Autodesk Inventor part; units mm, degrees
(part 4 of 6)
  line L918 (-92.1365, -59.7341) -> (-92.1319, -59.6995) projected
  line L919 (-92.1319, -59.6995) -> (-92.1268, -59.6649) projected
  line L920 (-92.1268, -59.6649) -> (-92.121, -59.6305) projected
  line L921 (-92.121, -59.6305) -> (-92.1147, -59.5962) projected
  line L922 (-92.1147, -59.5962) -> (-92.1077, -59.562) projected
  line L923 (-92.1077, -59.562) -> (-92.1001, -59.5279) projected
  line L924 (-92.1001, -59.5279) -> (-92.092, -59.494) projected
  line L925 (-92.092, -59.494) -> (-92.0833, -59.4602) projected
  line L926 (-92.0833, -59.4602) -> (-92.0739, -59.4265) projected
  line L927 (-92.0739, -59.4265) -> (-92.064, -59.3931) projected
  line L928 (-92.064, -59.3931) -> (-92.0535, -59.3598) projected
  line L929 (-92.0535, -59.3598) -> (-92.0424, -59.3267) projected
  line L930 (-92.0424, -59.3267) -> (-92.0308, -59.2938) projected
  line L931 (-92.0308, -59.2938) -> (-92.0186, -59.2611) projected
  line L932 (-92.0186, -59.2611) -> (-92.0058, -59.2286) projected
  line L933 (-92.0058, -59.2286) -> (-91.9924, -59.1963) projected
  line L934 (-91.9924, -59.1963) -> (-91.9785, -59.1643) projected
  line L935 (-91.9785, -59.1643) -> (-91.964, -59.1326) projected
  line L936 (-91.964, -59.1326) -> (-91.949, -59.1011) projected
  line L937 (-91.949, -59.1011) -> (-91.9334, -59.0698) projected
  line L938 (-91.9334, -59.0698) -> (-91.9173, -59.0389) projected
  line L939 (-91.9173, -59.0389) -> (-91.9006, -59.0082) projected
  line L940 (-91.9006, -59.0082) -> (-91.8835, -58.9778) projected
  line L941 (-91.8835, -58.9778) -> (-91.8657, -58.9477) projected
  line L942 (-91.8657, -58.9477) -> (-91.8475, -58.918) projected
  line L943 (-91.8475, -58.918) -> (-91.8287, -58.8885) projected
  line L944 (-91.8287, -58.8885) -> (-91.8095, -58.8594) projected
  line L945 (-91.8095, -58.8594) -> (-91.7897, -58.8307) projected
  line L946 (-91.7897, -58.8307) -> (-91.7694, -58.8022) projected
  line L947 (-91.7694, -58.8022) -> (-91.7487, -58.7742) projected
  line L948 (-91.7487, -58.7742) -> (-91.7274, -58.7465) projected
  line L949 (-91.7274, -58.7465) -> (-91.7057, -58.7192) projected
  line L950 (-91.7057, -58.7192) -> (-91.6835, -58.6922) projected
  line L951 (-91.6835, -58.6922) -> (-91.6608, -58.6657) projected
  line L952 (-91.6608, -58.6657) -> (-91.6377, -58.6396) projected
  line L953 (-91.6377, -58.6396) -> (-91.6141, -58.6138) projected
  line L954 (-91.6141, -58.6138) -> (-91.5901, -58.5885) projected
  line L955 (-91.5901, -58.5885) -> (-91.5656, -58.5636) projected
  line L956 (-91.5656, -58.5636) -> (-91.5407, -58.5391) projected
  line L957 (-91.5407, -58.5391) -> (-91.5154, -58.5151) projected
  line L958 (-91.5154, -58.5151) -> (-91.4897, -58.4915) projected
  line L959 (-91.4897, -58.4915) -> (-91.4635, -58.4684) projected
  line L960 (-91.4635, -58.4684) -> (-91.437, -58.4457) projected
  line L961 (-91.437, -58.4457) -> (-91.41, -58.4235) projected
  line L962 (-91.41, -58.4235) -> (-91.3827, -58.4018) projected
  line L963 (-91.3827, -58.4018) -> (-91.355, -58.3805) projected
  line L964 (-91.355, -58.3805) -> (-91.327, -58.3598) projected
  line L965 (-91.327, -58.3598) -> (-91.2986, -58.3395) projected
  line L966 (-91.2986, -58.3395) -> (-91.2698, -58.3197) projected
  line L967 (-91.2698, -58.3197) -> (-91.2407, -58.3005) projected
  line L968 (-91.2407, -58.3005) -> (-91.2112, -58.2817) projected
  line L969 (-91.2112, -58.2817) -> (-91.1815, -58.2635) projected
  line L970 (-91.1815, -58.2635) -> (-91.1514, -58.2458) projected
  line L971 (-91.1514, -58.2458) -> (-91.121, -58.2286) projected
  line L972 (-91.121, -58.2286) -> (-91.0904, -58.2119) projected
  line L973 (-91.0904, -58.2119) -> (-91.0594, -58.1958) projected
  line L974 (-91.0594, -58.1958) -> (-91.0282, -58.1802) projected
  line L975 (-91.0282, -58.1802) -> (-90.9966, -58.1652) projected
  line L976 (-90.9966, -58.1652) -> (-90.9649, -58.1507) projected
  line L977 (-90.9649, -58.1507) -> (-90.9329, -58.1368) projected
  line L978 (-90.9329, -58.1368) -> (-90.9006, -58.1234) projected
  line L979 (-90.9006, -58.1234) -> (-90.8681, -58.1107) projected
  line L980 (-90.8681, -58.1107) -> (-90.8354, -58.0984) projected
  line L981 (-90.8354, -58.0984) -> (-90.8025, -58.0868) projected
  line L982 (-90.8025, -58.0868) -> (-90.7694, -58.0757) projected
  line L983 (-90.7694, -58.0757) -> (-90.7362, -58.0652) projected
  line L984 (-90.7362, -58.0652) -> (-90.7027, -58.0553) projected
  line L985 (-90.7027, -58.0553) -> (-90.669, -58.046) projected
  line L986 (-90.669, -58.046) -> (-90.6353, -58.0372) projected
  line L987 (-90.6353, -58.0372) -> (-90.6013, -58.0291) projected
  line L988 (-90.6013, -58.0291) -> (-90.5672, -58.0215) projected
  line L989 (-90.5672, -58.0215) -> (-90.533, -58.0146) projected
  line L990 (-90.533, -58.0146) -> (-90.4987, -58.0082) projected
  line L991 (-90.4987, -58.0082) -> (-90.4643, -58.0024) projected
  line L992 (-90.4643, -58.0024) -> (-90.4298, -57.9973) projected
  line L993 (-90.4298, -57.9973) -> (-90.3951, -57.9927) projected
  line L994 (-90.3951, -57.9927) -> (-90.3605, -57.9888) projected
  line L995 (-90.3605, -57.9888) -> (-90.3257, -57.9854) projected
  line L996 (-90.3257, -57.9854) -> (-90.2909, -57.9827) projected
  line L997 (-90.2909, -57.9827) -> (-90.2561, -57.9806) projected
  line L998 (-90.2561, -57.9806) -> (-90.2212, -57.979) projected
  line L999 (-90.2212, -57.979) -> (-90.1863, -57.9781) projected
  line L1000 (-90.1863, -57.9781) -> (-90.1514, -57.9778) projected
  line L1001 (-90.1514, -57.9778) -> (-90.1165, -57.9781) projected
  line L1002 (-90.1165, -57.9781) -> (-90.0816, -57.979) projected
  line L1003 (-90.0816, -57.979) -> (-90.0467, -57.9806) projected
  line L1004 (-90.0467, -57.9806) -> (-90.0119, -57.9827) projected
  line L1005 (-90.0119, -57.9827) -> (-89.9771, -57.9854) projected
  line L1006 (-89.9771, -57.9854) -> (-89.9424, -57.9888) projected
  line L1007 (-89.9424, -57.9888) -> (-89.9077, -57.9927) projected
  line L1008 (-89.9077, -57.9927) -> (-89.8731, -57.9973) projected
  line L1009 (-89.8731, -57.9973) -> (-89.8385, -58.0024) projected
  line L1010 (-89.8385, -58.0024) -> (-89.8041, -58.0082) projected
  line L1011 (-89.8041, -58.0082) -> (-89.7698, -58.0146) projected
  line L1012 (-89.7698, -58.0146) -> (-89.7356, -58.0215) projected
  line L1013 (-89.7356, -58.0215) -> (-89.7015, -58.0291) projected
  line L1014 (-89.7015, -58.0291) -> (-89.6676, -58.0372) projected
  line L1015 (-89.6676, -58.0372) -> (-89.6338, -58.046) projected
  line L1016 (-89.6338, -58.046) -> (-89.6001, -58.0553) projected
  line L1017 (-89.6001, -58.0553) -> (-89.5667, -58.0652) projected
  line L1018 (-89.5667, -58.0652) -> (-89.5334, -58.0757) projected
  line L1019 (-89.5334, -58.0757) -> (-89.5003, -58.0868) projected
  line L1020 (-89.5003, -58.0868) -> (-89.4674, -58.0984) projected
  line L1021 (-89.4674, -58.0984) -> (-89.4347, -58.1107) projected
  line L1022 (-89.4347, -58.1107) -> (-89.4022, -58.1234) projected
  line L1023 (-89.4022, -58.1234) -> (-89.3699, -58.1368) projected
  line L1024 (-89.3699, -58.1368) -> (-89.3379, -58.1507) projected
  line L1025 (-89.3379, -58.1507) -> (-89.3062, -58.1652) projected
  line L1026 (-89.3062, -58.1652) -> (-89.2747, -58.1802) projected
  line L1027 (-89.2747, -58.1802) -> (-89.2434, -58.1958) projected
  line L1028 (-89.2434, -58.1958) -> (-89.2125, -58.2119) projected
  line L1029 (-89.2125, -58.2119) -> (-89.1818, -58.2286) projected
  line L1030 (-89.1818, -58.2286) -> (-89.1514, -58.2458) projected
  line L1031 (-89.1514, -58.2458) -> (-89.1213, -58.2635) projected
  line L1032 (-89.1213, -58.2635) -> (-89.0916, -58.2817) projected
  line L1033 (-89.0916, -58.2817) -> (-89.0621, -58.3005) projected
  line L1034 (-89.0621, -58.3005) -> (-89.033, -58.3197) projected
  line L1035 (-89.033, -58.3197) -> (-89.0043, -58.3395) projected
  line L1036 (-89.0043, -58.3395) -> (-88.9758, -58.3598) projected
  line L1037 (-88.9758, -58.3598) -> (-88.9478, -58.3805) projected
  line L1038 (-88.9478, -58.3805) -> (-88.9201, -58.4018) projected
  line L1039 (-88.9201, -58.4018) -> (-88.8928, -58.4235) projected
  line L1040 (-88.8928, -58.4235) -> (-88.8658, -58.4457) projected
  line L1041 (-88.8658, -58.4457) -> (-88.8393, -58.4684) projected
  line L1042 (-88.8393, -58.4684) -> (-88.8132, -58.4915) projected
  line L1043 (-88.8132, -58.4915) -> (-88.7874, -58.5151) projected
  line L1044 (-88.7874, -58.5151) -> (-88.7621, -58.5391) projected
  line L1045 (-88.7621, -58.5391) -> (-88.7372, -58.5636) projected
  line L1046 (-88.7372, -58.5636) -> (-88.7127, -58.5885) projected
  line L1047 (-88.7127, -58.5885) -> (-88.6887, -58.6138) projected
  line L1048 (-88.6887, -58.6138) -> (-88.6651, -58.6396) projected
  line L1049 (-88.6651, -58.6396) -> (-88.642, -58.6657) projected
  line L1050 (-88.642, -58.6657) -> (-88.6193, -58.6922) projected
  line L1051 (-88.6193, -58.6922) -> (-88.5971, -58.7192) projected
  line L1052 (-88.5971, -58.7192) -> (-88.5754, -58.7465) projected
  line L1053 (-88.5754, -58.7465) -> (-88.5541, -58.7742) projected
  line L1054 (-88.5541, -58.7742) -> (-88.5334, -58.8022) projected
  line L1055 (-88.5334, -58.8022) -> (-88.5131, -58.8307) projected
  line L1056 (-88.5131, -58.8307) -> (-88.4933, -58.8594) projected
  line L1057 (-88.4933, -58.8594) -> (-88.4741, -58.8885) projected
  line L1058 (-88.4741, -58.8885) -> (-88.4553, -58.918) projected
  line L1059 (-88.4553, -58.918) -> (-88.4371, -58.9477) projected
  line L1060 (-88.4371, -58.9477) -> (-88.4194, -58.9778) projected
  line L1061 (-88.4194, -58.9778) -> (-88.4022, -59.0082) projected
  line L1062 (-88.4022, -59.0082) -> (-88.3855, -59.0389) projected
  line L1063 (-88.3855, -59.0389) -> (-88.3694, -59.0698) projected
  line L1064 (-88.3694, -59.0698) -> (-88.3538, -59.1011) projected
  line L1065 (-88.3538, -59.1011) -> (-88.3388, -59.1326) projected
  line L1066 (-88.3388, -59.1326) -> (-88.3243, -59.1643) projected
  line L1067 (-88.3243, -59.1643) -> (-88.3104, -59.1963) projected
  line L1068 (-88.3104, -59.1963) -> (-88.297, -59.2286) projected
  line L1069 (-88.297, -59.2286) -> (-88.2843, -59.2611) projected
  line L1070 (-88.2843, -59.2611) -> (-88.272, -59.2938) projected
  line L1071 (-88.272, -59.2938) -> (-88.2604, -59.3267) projected
  line L1072 (-88.2604, -59.3267) -> (-88.2493, -59.3598) projected
  line L1073 (-88.2493, -59.3598) -> (-88.2388, -59.3931) projected
  line L1074 (-88.2388, -59.3931) -> (-88.2289, -59.4265) projected
  line L1075 (-88.2289, -59.4265) -> (-88.2196, -59.4602) projected
  line L1076 (-88.2196, -59.4602) -> (-88.2108, -59.494) projected
  line L1077 (-88.2108, -59.494) -> (-88.2027, -59.5279) projected
  line L1078 (-88.2027, -59.5279) -> (-88.1951, -59.562) projected
  line L1079 (-88.1951, -59.562) -> (-88.1882, -59.5962) projected
  line L1080 (-88.1882, -59.5962) -> (-88.1818, -59.6305) projected
  line L1081 (-88.1818, -59.6305) -> (-88.176, -59.6649) projected
  line L1082 (-88.176, -59.6649) -> (-88.1709, -59.6995) projected
  line L1083 (-88.1709, -59.6995) -> (-88.1663, -59.7341) projected
  line L1084 (-88.1663, -59.7341) -> (-88.1624, -59.7688) projected
  line L1085 (-88.1624, -59.7688) -> (-88.159, -59.8035) projected
  line L1086 (-88.159, -59.8035) -> (-88.1563, -59.8383) projected
  line L1087 (-88.1563, -59.8383) -> (-88.1542, -59.8731) projected
  line L1088 (-88.1542, -59.8731) -> (-88.1526, -59.908) projected
  line L1089 (-88.1526, -59.908) -> (-88.1517, -59.9429) projected
  line L1090 (-88.1517, -59.9429) -> (-88.1514, -59.9778) projected
  line L1091 (-88.1563, 60.1617) -> (-88.1542, 60.1269) projected
  line L1092 (-88.1542, 60.1269) -> (-88.1526, 60.092) projected
  line L1093 (-88.1526, 60.092) -> (-88.1517, 60.0571) projected
  line L1094 (-88.1517, 60.0571) -> (-88.1514, 60.0222) projected
  line L1095 (-88.1514, 60.0222) -> (-88.1517, 59.9873) projected
  line L1096 (-88.1517, 59.9873) -> (-88.1526, 59.9524) projected
  line L1097 (-88.1526, 59.9524) -> (-88.1542, 59.9175) projected
  line L1098 (-88.1542, 59.9175) -> (-88.1563, 59.8827) projected
  line L1099 (-88.1563, 59.8827) -> (-88.159, 59.8479) projected
  line L1100 (-88.159, 59.8479) -> (-88.1624, 59.8131) projected
  line L1101 (-88.1624, 59.8131) -> (-88.1663, 59.7785) projected
  line L1102 (-88.1663, 59.7785) -> (-88.1709, 59.7439) projected
  line L1103 (-88.1709, 59.7439) -> (-88.176, 59.7093) projected
  line L1104 (-88.176, 59.7093) -> (-88.1818, 59.6749) projected
  line L1105 (-88.1818, 59.6749) -> (-88.1882, 59.6406) projected
  line L1106 (-88.1882, 59.6406) -> (-88.1951, 59.6064) projected
  line L1107 (-88.1951, 59.6064) -> (-88.2027, 59.5723) projected
  line L1108 (-88.2027, 59.5723) -> (-88.2108, 59.5384) projected
  line L1109 (-88.2108, 59.5384) -> (-88.2196, 59.5046) projected
  line L1110 (-88.2196, 59.5046) -> (-88.2289, 59.4709) projected
  line L1111 (-88.2289, 59.4709) -> (-88.2388, 59.4375) projected
  line L1112 (-88.2388, 59.4375) -> (-88.2493, 59.4042) projected
  line L1113 (-88.2493, 59.4042) -> (-88.2604, 59.3711) projected
  line L1114 (-88.2604, 59.3711) -> (-88.272, 59.3382) projected
  line L1115 (-88.272, 59.3382) -> (-88.2843, 59.3055) projected
  line L1116 (-88.2843, 59.3055) -> (-88.297, 59.273) projected
  line L1117 (-88.297, 59.273) -> (-88.3104, 59.2407) projected
  line L1118 (-88.3104, 59.2407) -> (-88.3243, 59.2087) projected
  line L1119 (-88.3243, 59.2087) -> (-88.3388, 59.177) projected
  line L1120 (-88.3388, 59.177) -> (-88.3538, 59.1455) projected
  line L1121 (-88.3538, 59.1455) -> (-88.3694, 59.1142) projected
  line L1122 (-88.3694, 59.1142) -> (-88.3855, 59.0833) projected
  line L1123 (-88.3855, 59.0833) -> (-88.4022, 59.0526) projected
  line L1124 (-88.4022, 59.0526) -> (-88.4194, 59.0222) projected
  line L1125 (-88.4194, 59.0222) -> (-88.4371, 58.9921) projected
  line L1126 (-88.4371, 58.9921) -> (-88.4553, 58.9624) projected
  line L1127 (-88.4553, 58.9624) -> (-88.4741, 58.9329) projected
  line L1128 (-88.4741, 58.9329) -> (-88.4933, 58.9038) projected
  line L1129 (-88.4933, 58.9038) -> (-88.5131, 58.8751) projected
  line L1130 (-88.5131, 58.8751) -> (-88.5334, 58.8466) projected
  line L1131 (-88.5334, 58.8466) -> (-88.5541, 58.8186) projected
  line L1132 (-88.5541, 58.8186) -> (-88.5754, 58.7909) projected
  line L1133 (-88.5754, 58.7909) -> (-88.5971, 58.7636) projected
  line L1134 (-88.5971, 58.7636) -> (-88.6193, 58.7366) projected
  line L1135 (-88.6193, 58.7366) -> (-88.642, 58.7101) projected
  line L1136 (-88.642, 58.7101) -> (-88.6651, 58.6839) projected
  line L1137 (-88.6651, 58.6839) -> (-88.6887, 58.6582) projected
  line L1138 (-88.6887, 58.6582) -> (-88.7127, 58.6329) projected
  line L1139 (-88.7127, 58.6329) -> (-88.7372, 58.608) projected
  line L1140 (-88.7372, 58.608) -> (-88.7621, 58.5835) projected
  line L1141 (-88.7621, 58.5835) -> (-88.7874, 58.5595) projected
  line L1142 (-88.7874, 58.5595) -> (-88.8132, 58.5359) projected
  line L1143 (-88.8132, 58.5359) -> (-88.8393, 58.5128) projected
  line L1144 (-88.8393, 58.5128) -> (-88.8658, 58.4901) projected
  line L1145 (-88.8658, 58.4901) -> (-88.8928, 58.4679) projected
  line L1146 (-88.8928, 58.4679) -> (-88.9201, 58.4462) projected
  line L1147 (-88.9201, 58.4462) -> (-88.9478, 58.4249) projected
  line L1148 (-88.9478, 58.4249) -> (-88.9758, 58.4042) projected
  line L1149 (-88.9758, 58.4042) -> (-89.0043, 58.3839) projected
  line L1150 (-89.0043, 58.3839) -> (-89.033, 58.3641) projected
  line L1151 (-89.033, 58.3641) -> (-89.0621, 58.3449) projected
  line L1152 (-89.0621, 58.3449) -> (-89.0916, 58.3261) projected
  line L1153 (-89.0916, 58.3261) -> (-89.1213, 58.3079) projected
  line L1154 (-89.1213, 58.3079) -> (-89.1514, 58.2902) projected
  line L1155 (-89.1514, 58.2902) -> (-89.1818, 58.273) projected
  line L1156 (-89.1818, 58.273) -> (-89.2125, 58.2563) projected
  line L1157 (-89.2125, 58.2563) -> (-89.2434, 58.2402) projected
  line L1158 (-89.2434, 58.2402) -> (-89.2747, 58.2246) projected
  line L1159 (-89.2747, 58.2246) -> (-89.3062, 58.2096) projected
  line L1160 (-89.3062, 58.2096) -> (-89.3379, 58.1951) projected
  line L1161 (-89.3379, 58.1951) -> (-89.3699, 58.1812) projected
  line L1162 (-89.3699, 58.1812) -> (-89.4022, 58.1678) projected
  line L1163 (-89.4022, 58.1678) -> (-89.4347, 58.155) projected
  line L1164 (-89.4347, 58.155) -> (-89.4674, 58.1428) projected
  line L1165 (-89.4674, 58.1428) -> (-89.5003, 58.1312) projected
  line L1166 (-89.5003, 58.1312) -> (-89.5334, 58.1201) projected
  line L1167 (-89.5334, 58.1201) -> (-89.5667, 58.1096) projected
  line L1168 (-89.5667, 58.1096) -> (-89.6001, 58.0997) projected
  line L1169 (-89.6001, 58.0997) -> (-89.6338, 58.0904) projected
  line L1170 (-89.6338, 58.0904) -> (-89.6676, 58.0816) projected
  line L1171 (-89.6676, 58.0816) -> (-89.7015, 58.0735) projected
  line L1172 (-89.7015, 58.0735) -> (-89.7356, 58.0659) projected
  line L1173 (-89.7356, 58.0659) -> (-89.7698, 58.059) projected
  line L1174 (-89.7698, 58.059) -> (-89.8041, 58.0526) projected
  line L1175 (-89.8041, 58.0526) -> (-89.8385, 58.0468) projected
  line L1176 (-89.8385, 58.0468) -> (-89.8731, 58.0417) projected
  line L1177 (-89.8731, 58.0417) -> (-89.9077, 58.0371) projected
  line L1178 (-89.9077, 58.0371) -> (-89.9424, 58.0332) projected
  line L1179 (-89.9424, 58.0332) -> (-89.9771, 58.0298) projected
  line L1180 (-89.9771, 58.0298) -> (-90.0119, 58.0271) projected
  line L1181 (-90.0119, 58.0271) -> (-90.0467, 58.0249) projected
  line L1182 (-90.0467, 58.0249) -> (-90.0816, 58.0234) projected
  line L1183 (-90.0816, 58.0234) -> (-90.1165, 58.0225) projected
  line L1184 (-90.1165, 58.0225) -> (-90.1514, 58.0222) projected
  line L1185 (-90.1514, 58.0222) -> (-90.1863, 58.0225) projected
  line L1186 (-90.1863, 58.0225) -> (-90.2212, 58.0234) projected
  line L1187 (-90.2212, 58.0234) -> (-90.2561, 58.0249) projected
  line L1188 (-90.2561, 58.0249) -> (-90.2909, 58.0271) projected
  line L1189 (-90.2909, 58.0271) -> (-90.3257, 58.0298) projected
  line L1190 (-90.3257, 58.0298) -> (-90.3605, 58.0332) projected
  line L1191 (-90.3605, 58.0332) -> (-90.3951, 58.0371) projected
  line L1192 (-90.3951, 58.0371) -> (-90.4298, 58.0417) projected
  line L1193 (-90.4298, 58.0417) -> (-90.4643, 58.0468) projected
  line L1194 (-90.4643, 58.0468) -> (-90.4987, 58.0526) projected
  line L1195 (-90.4987, 58.0526) -> (-90.533, 58.059) projected
  line L1196 (-90.533, 58.059) -> (-90.5672, 58.0659) projected
  line L1197 (-90.5672, 58.0659) -> (-90.6013, 58.0735) projected
  line L1198 (-90.6013, 58.0735) -> (-90.6353, 58.0816) projected
  line L1199 (-90.6353, 58.0816) -> (-90.669, 58.0904) projected
  line L1200 (-90.669, 58.0904) -> (-90.7027, 58.0997) projected
  line L1201 (-90.7027, 58.0997) -> (-90.7362, 58.1096) projected
  line L1202 (-90.7362, 58.1096) -> (-90.7694, 58.1201) projected
  line L1203 (-90.7694, 58.1201) -> (-90.8025, 58.1312) projected
  line L1204 (-90.8025, 58.1312) -> (-90.8354, 58.1428) projected
  line L1205 (-90.8354, 58.1428) -> (-90.8681, 58.155) projected
  line L1206 (-90.8681, 58.155) -> (-90.9006, 58.1678) projected
  line L1207 (-90.9006, 58.1678) -> (-90.9329, 58.1812) projected
  line L1208 (-90.9329, 58.1812) -> (-90.9649, 58.1951) projected
  line L1209 (-90.9649, 58.1951) -> (-90.9966, 58.2096) projected
  line L1210 (-90.9966, 58.2096) -> (-91.0282, 58.2246) projected
  line L1211 (-91.0282, 58.2246) -> (-91.0594, 58.2402) projected
  line L1212 (-91.0594, 58.2402) -> (-91.0904, 58.2563) projected
  line L1213 (-91.0904, 58.2563) -> (-91.121, 58.273) projected
  line L1214 (-91.121, 58.273) -> (-91.1514, 58.2902) projected
  line L1215 (-91.1514, 58.2902) -> (-91.1815, 58.3079) projected
  line L1216 (-91.1815, 58.3079) -> (-91.2112, 58.3261) projected
  line L1217 (-91.2112, 58.3261) -> (-91.2407, 58.3449) projected
  line L1218 (-91.2407, 58.3449) -> (-91.2698, 58.3641) projected
  line L1219 (-91.2698, 58.3641) -> (-91.2986, 58.3839) projected
  line L1220 (-91.2986, 58.3839) -> (-91.327, 58.4042) projected
  line L1221 (-91.327, 58.4042) -> (-91.355, 58.4249) projected
  line L1222 (-91.355, 58.4249) -> (-91.3827, 58.4462) projected
  line L1223 (-91.3827, 58.4462) -> (-91.41, 58.4679) projected
  line L1224 (-91.41, 58.4679) -> (-91.437, 58.4901) projected
  line L1225 (-91.437, 58.4901) -> (-91.4635, 58.5128) projected
  line L1226 (-91.4635, 58.5128) -> (-91.4897, 58.5359) projected
  line L1227 (-91.4897, 58.5359) -> (-91.5154, 58.5595) projected
  line L1228 (-91.5154, 58.5595) -> (-91.5407, 58.5835) projected
  line L1229 (-91.5407, 58.5835) -> (-91.5656, 58.608) projected
  line L1230 (-91.5656, 58.608) -> (-91.5901, 58.6329) projected
  line L1231 (-91.5901, 58.6329) -> (-91.6141, 58.6582) projected
  line L1232 (-91.6141, 58.6582) -> (-91.6377, 58.6839) projected
  line L1233 (-91.6377, 58.6839) -> (-91.6608, 58.7101) projected
  line L1234 (-91.6608, 58.7101) -> (-91.6835, 58.7366) projected
  line L1235 (-91.6835, 58.7366) -> (-91.7057, 58.7636) projected
  line L1236 (-91.7057, 58.7636) -> (-91.7274, 58.7909) projected
  line L1237 (-91.7274, 58.7909) -> (-91.7487, 58.8186) projected
  line L1238 (-91.7487, 58.8186) -> (-91.7694, 58.8466) projected
  line L1239 (-91.7694, 58.8466) -> (-91.7897, 58.8751) projected
  line L1240 (-91.7897, 58.8751) -> (-91.8095, 58.9038) projected
  line L1241 (-91.8095, 58.9038) -> (-91.8287, 58.9329) projected
  line L1242 (-91.8287, 58.9329) -> (-91.8475, 58.9624) projected
  line L1243 (-91.8475, 58.9624) -> (-91.8657, 58.9921) projected
  line L1244 (-91.8657, 58.9921) -> (-91.8835, 59.0222) projected
  line L1245 (-91.8835, 59.0222) -> (-91.9006, 59.0526) projected
  line L1246 (-91.9006, 59.0526) -> (-91.9173, 59.0833) projected
  line L1247 (-91.9173, 59.0833) -> (-91.9334, 59.1142) projected
  line L1248 (-91.9334, 59.1142) -> (-91.949, 59.1455) projected
  line L1249 (-91.949, 59.1455) -> (-91.964, 59.177) projected
  line L1250 (-91.964, 59.177) -> (-91.9785, 59.2087) projected
  line L1251 (-91.9785, 59.2087) -> (-91.9924, 59.2407) projected
  line L1252 (-91.9924, 59.2407) -> (-92.0058, 59.273) projected
  line L1253 (-92.0058, 59.273) -> (-92.0186, 59.3055) projected
  line L1254 (-92.0186, 59.3055) -> (-92.0308, 59.3382) projected
  line L1255 (-92.0308, 59.3382) -> (-92.0424, 59.3711) projected
  line L1256 (-92.0424, 59.3711) -> (-92.0535, 59.4042) projected
  line L1257 (-92.0535, 59.4042) -> (-92.064, 59.4375) projected
  line L1258 (-92.064, 59.4375) -> (-92.0739, 59.4709) projected
  line L1259 (-92.0739, 59.4709) -> (-92.0833, 59.5046) projected
  line L1260 (-92.0833, 59.5046) -> (-92.092, 59.5384) projected
  line L1261 (-92.092, 59.5384) -> (-92.1001, 59.5723) projected
  line L1262 (-92.1001, 59.5723) -> (-92.1077, 59.6064) projected
  line L1263 (-92.1077, 59.6064) -> (-92.1147, 59.6406) projected
  line L1264 (-92.1147, 59.6406) -> (-92.121, 59.6749) projected
  line L1265 (-92.121, 59.6749) -> (-92.1268, 59.7093) projected
  line L1266 (-92.1268, 59.7093) -> (-92.1319, 59.7439) projected
  line L1267 (-92.1319, 59.7439) -> (-92.1365, 59.7785) projected
  line L1268 (-92.1365, 59.7785) -> (-92.1404, 59.8131) projected
  line L1269 (-92.1404, 59.8131) -> (-92.1438, 59.8479) projected
  line L1270 (-92.1438, 59.8479) -> (-92.1465, 59.8827) projected
  line L1271 (-92.1465, 59.8827) -> (-92.1487, 59.9175) projected
  line L1272 (-92.1487, 59.9175) -> (-92.1502, 59.9524) projected
  line L1273 (-92.1502, 59.9524) -> (-92.1511, 59.9873) projected
  line L1274 (-92.1511, 59.9873) -> (-92.1514, 60.0222) projected
  line L1275 (-92.1514, 60.0222) -> (-92.1511, 60.0571) projected
  line L1276 (-92.1511, 60.0571) -> (-92.1502, 60.092) projected
  line L1277 (-92.1502, 60.092) -> (-92.1487, 60.1269) projected
  line L1278 (-92.1487, 60.1269) -> (-92.1465, 60.1617) projected
  line L1279 (-92.1465, 60.1617) -> (-92.1438, 60.1965) projected
  line L1280 (-92.1438, 60.1965) -> (-92.1404, 60.2313) projected
  line L1281 (-92.1404, 60.2313) -> (-92.1365, 60.2659) projected
  line L1282 (-92.1365, 60.2659) -> (-92.1319, 60.3005) projected
  line L1283 (-92.1319, 60.3005) -> (-92.1268, 60.3351) projected
  line L1284 (-92.1268, 60.3351) -> (-92.121, 60.3695) projected
  line L1285 (-92.121, 60.3695) -> (-92.1147, 60.4038) projected
  line L1286 (-92.1147, 60.4038) -> (-92.1077, 60.438) projected
  line L1287 (-92.1077, 60.438) -> (-92.1001, 60.4721) projected
  line L1288 (-92.1001, 60.4721) -> (-92.092, 60.506) projected
  line L1289 (-92.092, 60.506) -> (-92.0833, 60.5398) projected
  line L1290 (-92.0833, 60.5398) -> (-92.0739, 60.5735) projected
  line L1291 (-92.0739, 60.5735) -> (-92.064, 60.6069) projected
  line L1292 (-92.064, 60.6069) -> (-92.0535, 60.6402) projected
  line L1293 (-92.0535, 60.6402) -> (-92.0424, 60.6733) projected
  line L1294 (-92.0424, 60.6733) -> (-92.0308, 60.7062) projected
  line L1295 (-92.0308, 60.7062) -> (-92.0186, 60.7389) projected
  line L1296 (-92.0186, 60.7389) -> (-92.0058, 60.7714) projected
  line L1297 (-92.0058, 60.7714) -> (-91.9924, 60.8037) projected
  line L1298 (-91.9924, 60.8037) -> (-91.9785, 60.8357) projected
  line L1299 (-91.9785, 60.8357) -> (-91.964, 60.8674) projected
  line L1300 (-91.964, 60.8674) -> (-91.949, 60.8989) projected
  line L1301 (-91.949, 60.8989) -> (-91.9334, 60.9302) projected
  line L1302 (-91.9334, 60.9302) -> (-91.9173, 60.9611) projected
  line L1303 (-91.9173, 60.9611) -> (-91.9006, 60.9918) projected
  line L1304 (-91.9006, 60.9918) -> (-91.8835, 61.0222) projected
  line L1305 (-91.8835, 61.0222) -> (-91.8657, 61.0523) projected
  line L1306 (-91.8657, 61.0523) -> (-91.8475, 61.082) projected
  line L1307 (-91.8475, 61.082) -> (-91.8287, 61.1115) projected
  line L1308 (-91.8287, 61.1115) -> (-91.8095, 61.1406) projected
  line L1309 (-91.8095, 61.1406) -> (-91.7897, 61.1694) projected
  line L1310 (-91.7897, 61.1694) -> (-91.7694, 61.1978) projected
  line L1311 (-91.7694, 61.1978) -> (-91.7487, 61.2258) projected
  line L1312 (-91.7487, 61.2258) -> (-91.7274, 61.2535) projected
  line L1313 (-91.7274, 61.2535) -> (-91.7057, 61.2808) projected
  line L1314 (-91.7057, 61.2808) -> (-91.6835, 61.3078) projected
  line L1315 (-91.6835, 61.3078) -> (-91.6608, 61.3343) projected
  line L1316 (-91.6608, 61.3343) -> (-91.6377, 61.3605) projected
  line L1317 (-91.6377, 61.3605) -> (-91.6141, 61.3862) projected
  line L1318 (-91.6141, 61.3862) -> (-91.5901, 61.4115) projected
  line L1319 (-91.5901, 61.4115) -> (-91.5656, 61.4364) projected
  line L1320 (-91.5656, 61.4364) -> (-91.5407, 61.4609) projected
  line L1321 (-91.5407, 61.4609) -> (-91.5154, 61.4849) projected
  line L1322 (-91.5154, 61.4849) -> (-91.4897, 61.5085) projected
  line L1323 (-91.4897, 61.5085) -> (-91.4635, 61.5316) projected
  line L1324 (-91.4635, 61.5316) -> (-91.437, 61.5543) projected
  line L1325 (-91.437, 61.5543) -> (-91.41, 61.5765) projected
  line L1326 (-91.41, 61.5765) -> (-91.3827, 61.5982) projected
  line L1327 (-91.3827, 61.5982) -> (-91.355, 61.6195) projected
  line L1328 (-91.355, 61.6195) -> (-91.327, 61.6402) projected
  line L1329 (-91.327, 61.6402) -> (-91.2986, 61.6605) projected
  line L1330 (-91.2986, 61.6605) -> (-91.2698, 61.6803) projected
  line L1331 (-91.2698, 61.6803) -> (-91.2407, 61.6995) projected
  line L1332 (-91.2407, 61.6995) -> (-91.2112, 61.7183) projected
  line L1333 (-91.2112, 61.7183) -> (-91.1815, 61.7365) projected
  line L1334 (-91.1815, 61.7365) -> (-91.1514, 61.7543) projected
  line L1335 (-91.1514, 61.7543) -> (-91.121, 61.7714) projected
  line L1336 (-91.121, 61.7714) -> (-91.0904, 61.7881) projected
  line L1337 (-91.0904, 61.7881) -> (-91.0594, 61.8042) projected
  line L1338 (-91.0594, 61.8042) -> (-91.0282, 61.8198) projected
  line L1339 (-91.0282, 61.8198) -> (-90.9966, 61.8348) projected
  line L1340 (-90.9966, 61.8348) -> (-90.9649, 61.8493) projected
  line L1341 (-90.9649, 61.8493) -> (-90.9329, 61.8632) projected
  line L1342 (-90.9329, 61.8632) -> (-90.9006, 61.8766) projected
  line L1343 (-90.9006, 61.8766) -> (-90.8681, 61.8894) projected
  line L1344 (-90.8681, 61.8894) -> (-90.8354, 61.9016) projected
  line L1345 (-90.8354, 61.9016) -> (-90.8025, 61.9132) projected
  line L1346 (-90.8025, 61.9132) -> (-90.7694, 61.9243) projected
  line L1347 (-90.7694, 61.9243) -> (-90.7362, 61.9348) projected
  line L1348 (-90.7362, 61.9348) -> (-90.7027, 61.9447) projected
  line L1349 (-90.7027, 61.9447) -> (-90.669, 61.9541) projected
  line L1350 (-90.669, 61.9541) -> (-90.6353, 61.9628) projected
  line L1351 (-90.6353, 61.9628) -> (-90.6013, 61.9709) projected
  line L1352 (-90.6013, 61.9709) -> (-90.5672, 61.9785) projected
  line L1353 (-90.5672, 61.9785) -> (-90.533, 61.9855) projected
  line L1354 (-90.533, 61.9855) -> (-90.4987, 61.9918) projected
  line L1355 (-90.4987, 61.9918) -> (-90.4643, 61.9976) projected
  line L1356 (-90.4643, 61.9976) -> (-90.4298, 62.0027) projected
  line L1357 (-90.4298, 62.0027) -> (-90.3951, 62.0073) projected
  line L1358 (-90.3951, 62.0073) -> (-90.3605, 62.0112) projected
  line L1359 (-90.3605, 62.0112) -> (-90.3257, 62.0146) projected
  line L1360 (-90.3257, 62.0146) -> (-90.2909, 62.0173) projected
  line L1361 (-90.2909, 62.0173) -> (-90.2561, 62.0195) projected
  line L1362 (-90.2561, 62.0195) -> (-90.2212, 62.021) projected
  line L1363 (-90.2212, 62.021) -> (-90.1863, 62.0219) projected
  line L1364 (-90.1863, 62.0219) -> (-90.1514, 62.0222) projected
  line L1365 (-90.1514, 62.0222) -> (-90.1165, 62.0219) projected
  line L1366 (-90.1165, 62.0219) -> (-90.0816, 62.021) projected
  line L1367 (-90.0816, 62.021) -> (-90.0467, 62.0195) projected
  line L1368 (-90.0467, 62.0195) -> (-90.0119, 62.0173) projected
  line L1369 (-90.0119, 62.0173) -> (-89.9771, 62.0146) projected
  line L1370 (-89.9771, 62.0146) -> (-89.9424, 62.0112) projected
  line L1371 (-89.9424, 62.0112) -> (-89.9077, 62.0073) projected
  line L1372 (-89.9077, 62.0073) -> (-89.8731, 62.0027) projected
  line L1373 (-89.8731, 62.0027) -> (-89.8385, 61.9976) projected
  line L1374 (-89.8385, 61.9976) -> (-89.8041, 61.9918) projected
  line L1375 (-89.8041, 61.9918) -> (-89.7698, 61.9855) projected
  line L1376 (-89.7698, 61.9855) -> (-89.7356, 61.9785) projected
  line L1377 (-89.7356, 61.9785) -> (-89.7015, 61.9709) projected
  line L1378 (-89.7015, 61.9709) -> (-89.6676, 61.9628) projected
  line L1379 (-89.6676, 61.9628) -> (-89.6338, 61.9541) projected
  line L1380 (-89.6338, 61.9541) -> (-89.6001, 61.9447) projected
  line L1381 (-89.6001, 61.9447) -> (-89.5667, 61.9348) projected
  line L1382 (-89.5667, 61.9348) -> (-89.5334, 61.9243) projected
  line L1383 (-89.5334, 61.9243) -> (-89.5003, 61.9132) projected
  line L1384 (-89.5003, 61.9132) -> (-89.4674, 61.9016) projected
  line L1385 (-89.4674, 61.9016) -> (-89.4347, 61.8894) projected
  line L1386 (-89.4347, 61.8894) -> (-89.4022, 61.8766) projected
  line L1387 (-89.4022, 61.8766) -> (-89.3699, 61.8632) projected
  line L1388 (-89.3699, 61.8632) -> (-89.3379, 61.8493) projected
  line L1389 (-89.3379, 61.8493) -> (-89.3062, 61.8348) projected
  line L1390 (-89.3062, 61.8348) -> (-89.2747, 61.8198) projected
  line L1391 (-89.2747, 61.8198) -> (-89.2434, 61.8042) projected
  line L1392 (-89.2434, 61.8042) -> (-89.2125, 61.7881) projected
  line L1393 (-89.2125, 61.7881) -> (-89.1818, 61.7714) projected
  line L1394 (-89.1818, 61.7714) -> (-89.1514, 61.7543) projected
  line L1395 (-89.1514, 61.7543) -> (-89.1213, 61.7365) projected
  line L1396 (-89.1213, 61.7365) -> (-89.0916, 61.7183) projected
  line L1397 (-89.0916, 61.7183) -> (-89.0621, 61.6995) projected
  line L1398 (-89.0621, 61.6995) -> (-89.033, 61.6803) projected
  line L1399 (-89.033, 61.6803) -> (-89.0043, 61.6605) projected
  line L1400 (-89.0043, 61.6605) -> (-88.9758, 61.6402) projected
  line L1401 (-88.9758, 61.6402) -> (-88.9478, 61.6195) projected
  line L1402 (-88.9478, 61.6195) -> (-88.9201, 61.5982) projected
  line L1403 (-88.9201, 61.5982) -> (-88.8928, 61.5765) projected
  line L1404 (-88.8928, 61.5765) -> (-88.8658, 61.5543) projected
  line L1405 (-88.8658, 61.5543) -> (-88.8393, 61.5316) projected
  line L1406 (-88.8393, 61.5316) -> (-88.8132, 61.5085) projected
  line L1407 (-88.8132, 61.5085) -> (-88.7874, 61.4849) projected
  line L1408 (-88.7874, 61.4849) -> (-88.7621, 61.4609) projected
  line L1409 (-88.7621, 61.4609) -> (-88.7372, 61.4364) projected
  line L1410 (-88.7372, 61.4364) -> (-88.7127, 61.4115) projected
  line L1411 (-88.7127, 61.4115) -> (-88.6887, 61.3862) projected
  line L1412 (-88.6887, 61.3862) -> (-88.6651, 61.3605) projected
  line L1413 (-88.6651, 61.3605) -> (-88.642, 61.3343) projected
  line L1414 (-88.642, 61.3343) -> (-88.6193, 61.3078) projected
  line L1415 (-88.6193, 61.3078) -> (-88.5971, 61.2808) projected
  line L1416 (-88.5971, 61.2808) -> (-88.5754, 61.2535) projected
  line L1417 (-88.5754, 61.2535) -> (-88.5541, 61.2258) projected
  line L1418 (-88.5541, 61.2258) -> (-88.5334, 61.1978) projected
  line L1419 (-88.5334, 61.1978) -> (-88.5131, 61.1694) projected
  line L1420 (-88.5131, 61.1694) -> (-88.4933, 61.1406) projected
  line L1421 (-88.4933, 61.1406) -> (-88.4741, 61.1115) projected
  line L1422 (-88.4741, 61.1115) -> (-88.4553, 61.082) projected
  line L1423 (-88.4553, 61.082) -> (-88.4371, 61.0523) projected
  line L1424 (-88.4371, 61.0523) -> (-88.4194, 61.0222) projected
  line L1425 (-88.4194, 61.0222) -> (-88.4022, 60.9918) projected
  line L1426 (-88.4022, 60.9918) -> (-88.3855, 60.9611) projected
  line L1427 (-88.3855, 60.9611) -> (-88.3694, 60.9302) projected
  line L1428 (-88.3694, 60.9302) -> (-88.3538, 60.8989) projected
  line L1429 (-88.3538, 60.8989) -> (-88.3388, 60.8674) projected
  line L1430 (-88.3388, 60.8674) -> (-88.3243, 60.8357) projected
  line L1431 (-88.3243, 60.8357) -> (-88.3104, 60.8037) projected
  line L1432 (-88.3104, 60.8037) -> (-88.297, 60.7714) projected
  line L1433 (-88.297, 60.7714) -> (-88.2843, 60.7389) projected
  line L1434 (-88.2843, 60.7389) -> (-88.272, 60.7062) projected
  line L1435 (-88.272, 60.7062) -> (-88.2604, 60.6733) projected
  line L1436 (-88.2604, 60.6733) -> (-88.2493, 60.6402) projected
  line L1437 (-88.2493, 60.6402) -> (-88.2388, 60.6069) projected
  line L1438 (-88.2388, 60.6069) -> (-88.2289, 60.5735) projected
  line L1439 (-88.2289, 60.5735) -> (-88.2196, 60.5398) projected
  line L1440 (-88.2196, 60.5398) -> (-88.2108, 60.506) projected
  line L1441 (-88.2108, 60.506) -> (-88.2027, 60.4721) projected
  line L1442 (-88.2027, 60.4721) -> (-88.1951, 60.438) projected
  line L1443 (-88.1951, 60.438) -> (-88.1882, 60.4038) projected
  line L1444 (-88.1882, 60.4038) -> (-88.1818, 60.3695) projected
  line L1445 (-88.1818, 60.3695) -> (-88.176, 60.3351) projected
  line L1446 (-88.176, 60.3351) -> (-88.1709, 60.3005) projected
  line L1447 (-88.1709, 60.3005) -> (-88.1663, 60.2659) projected
  line L1448 (-88.1663, 60.2659) -> (-88.1624, 60.2313) projected
  line L1449 (-88.1624, 60.2313) -> (-88.159, 60.1965) projected
  line L1450 (-88.159, 60.1965) -> (-88.1563, 60.1617) projected
  line L1451 (94.8475, 65.0222) -> (-95.1577, 65.0222) projected
  line L1452 (94.8475, -64.9778) -> (94.8475, 65.0222) projected
  line L1453 (94.8475, 65.0222) -> (-95.1577, 65.0222) projected
  line L1454 (-95.1577, 65.0222) -> (-95.1577, -64.9778) projected
  line L1455 (-95.1577, -64.9778) -> (94.8475, -64.9778) projected
  line L1456 (91.8485, 60.0222) -> (91.8482, 59.9873) projected
  line L1457 (91.8482, 59.9873) -> (91.8473, 59.9524) projected
  line L1458 (91.8473, 59.9524) -> (91.8457, 59.9175) projected
  line L1459 (91.8457, 59.9175) -> (91.8436, 59.8827) projected
  line L1460 (91.8436, 59.8827) -> (91.8409, 59.8479) projected
  line L1461 (91.8409, 59.8479) -> (91.8375, 59.8131) projected
  line L1462 (91.8375, 59.8131) -> (91.8336, 59.7785) projected
  line L1463 (91.8336, 59.7785) -> (91.829, 59.7439) projected
  line L1464 (91.829, 59.7439) -> (91.8239, 59.7093) projected
  line L1465 (91.8239, 59.7093) -> (91.8181, 59.6749) projected
  line L1466 (91.8181, 59.6749) -> (91.8117, 59.6406) projected
  line L1467 (91.8117, 59.6406) -> (91.8048, 59.6064) projected
  line L1468 (91.8048, 59.6064) -> (91.7972, 59.5723) projected
  line L1469 (91.7972, 59.5723) -> (91.7891, 59.5384) projected
  line L1470 (91.7891, 59.5384) -> (91.7803, 59.5046) projected
  line L1471 (91.7803, 59.5046) -> (91.771, 59.4709) projected
  line L1472 (91.771, 59.4709) -> (91.7611, 59.4375) projected
  line L1473 (91.7611, 59.4375) -> (91.7506, 59.4042) projected
  line L1474 (91.7506, 59.4042) -> (91.7395, 59.3711) projected
  line L1475 (91.7395, 59.3711) -> (91.7279, 59.3382) projected
  line L1476 (91.7279, 59.3382) -> (91.7156, 59.3055) projected
  line L1477 (91.7156, 59.3055) -> (91.7028, 59.273) projected
  line L1478 (91.7028, 59.273) -> (91.6895, 59.2407) projected
  line L1479 (91.6895, 59.2407) -> (91.6756, 59.2087) projected
  line L1480 (91.6756, 59.2087) -> (91.6611, 59.177) projected
  line L1481 (91.6611, 59.177) -> (91.6461, 59.1455) projected
  line L1482 (91.6461, 59.1455) -> (91.6305, 59.1142) projected
  line L1483 (91.6305, 59.1142) -> (91.6144, 59.0833) projected
  line L1484 (91.6144, 59.0833) -> (91.5977, 59.0526) projected
  line L1485 (91.5977, 59.0526) -> (91.5805, 59.0222) projected
  line L1486 (91.5805, 59.0222) -> (91.5628, 58.9921) projected
  line L1487 (91.5628, 58.9921) -> (91.5446, 58.9624) projected
  line L1488 (91.5446, 58.9624) -> (91.5258, 58.9329) projected
  line L1489 (91.5258, 58.9329) -> (91.5066, 58.9038) projected
  line L1490 (91.5066, 58.9038) -> (91.4868, 58.8751) projected
  line L1491 (91.4868, 58.8751) -> (91.4665, 58.8466) projected
  line L1492 (91.4665, 58.8466) -> (91.4458, 58.8186) projected
  line L1493 (91.4458, 58.8186) -> (91.4245, 58.7909) projected
  line L1494 (91.4245, 58.7909) -> (91.4028, 58.7636) projected
  line L1495 (91.4028, 58.7636) -> (91.3806, 58.7366) projected
  line L1496 (91.3806, 58.7366) -> (91.3579, 58.7101) projected
  line L1497 (91.3579, 58.7101) -> (91.3348, 58.6839) projected
  line L1498 (91.3348, 58.6839) -> (91.3112, 58.6582) projected
  line L1499 (91.3112, 58.6582) -> (91.2872, 58.6329) projected
  line L1500 (91.2872, 58.6329) -> (91.2627, 58.608) projected
  line L1501 (91.2627, 58.608) -> (91.2378, 58.5835) projected
  line L1502 (91.2378, 58.5835) -> (91.2125, 58.5595) projected
  line L1503 (91.2125, 58.5595) -> (91.1867, 58.5359) projected
  line L1504 (91.1867, 58.5359) -> (91.1606, 58.5128) projected
  line L1505 (91.1606, 58.5128) -> (91.1341, 58.4901) projected
  line L1506 (91.1341, 58.4901) -> (91.1071, 58.4679) projected
  line L1507 (91.1071, 58.4679) -> (91.0798, 58.4462) projected
  line L1508 (91.0798, 58.4462) -> (91.0521, 58.4249) projected
  line L1509 (91.0521, 58.4249) -> (91.0241, 58.4042) projected
  line L1510 (91.0241, 58.4042) -> (90.9956, 58.3839) projected
  line L1511 (90.9956, 58.3839) -> (90.9669, 58.3641) projected
  line L1512 (90.9669, 58.3641) -> (90.9378, 58.3449) projected
  line L1513 (90.9378, 58.3449) -> (90.9083, 58.3261) projected
  line L1514 (90.9083, 58.3261) -> (90.8786, 58.3079) projected
  line L1515 (90.8786, 58.3079) -> (90.8485, 58.2902) projected
  line L1516 (90.8485, 58.2902) -> (90.8181, 58.273) projected
  line L1517 (90.8181, 58.273) -> (90.7874, 58.2563) projected
  line L1518 (90.7874, 58.2563) -> (90.7565, 58.2402) projected
  line L1519 (90.7565, 58.2402) -> (90.7252, 58.2246) projected
  line L1520 (90.7252, 58.2246) -> (90.6937, 58.2096) projected
  line L1521 (90.6937, 58.2096) -> (90.662, 58.1951) projected
  line L1522 (90.662, 58.1951) -> (90.6299, 58.1812) projected
  line L1523 (90.6299, 58.1812) -> (90.5977, 58.1678) projected
  line L1524 (90.5977, 58.1678) -> (90.5652, 58.155) projected
  line L1525 (90.5652, 58.155) -> (90.5325, 58.1428) projected
  line L1526 (90.5325, 58.1428) -> (90.4996, 58.1312) projected
  line L1527 (90.4996, 58.1312) -> (90.4665, 58.1201) projected
  line L1528 (90.4665, 58.1201) -> (90.4332, 58.1096) projected
  line L1529 (90.4332, 58.1096) -> (90.3998, 58.0997) projected
  line L1530 (90.3998, 58.0997) -> (90.3661, 58.0904) projected
  line L1531 (90.3661, 58.0904) -> (90.3323, 58.0816) projected
  line L1532 (90.3323, 58.0816) -> (90.2984, 58.0735) projected
  line L1533 (90.2984, 58.0735) -> (90.2643, 58.0659) projected
  line L1534 (90.2643, 58.0659) -> (90.2301, 58.059) projected
  line L1535 (90.2301, 58.059) -> (90.1958, 58.0526) projected
  line L1536 (90.1958, 58.0526) -> (90.1614, 58.0468) projected
  line L1537 (90.1614, 58.0468) -> (90.1268, 58.0417) projected
  line L1538 (90.1268, 58.0417) -> (90.0922, 58.0371) projected
  line L1539 (90.0922, 58.0371) -> (90.0575, 58.0332) projected
  line L1540 (90.0575, 58.0332) -> (90.0228, 58.0298) projected
  line L1541 (90.0228, 58.0298) -> (89.988, 58.0271) projected
  line L1542 (89.988, 58.0271) -> (89.9532, 58.0249) projected
  line L1543 (89.9532, 58.0249) -> (89.9183, 58.0234) projected
  line L1544 (89.9183, 58.0234) -> (89.8834, 58.0225) projected
  line L1545 (89.8834, 58.0225) -> (89.8485, 58.0222) projected
  line L1546 (89.8485, 58.0222) -> (89.8136, 58.0225) projected
  line L1547 (89.8136, 58.0225) -> (89.7787, 58.0234) projected
  line L1548 (89.7787, 58.0234) -> (89.7438, 58.0249) projected
  line L1549 (89.7438, 58.0249) -> (89.709, 58.0271) projected
  line L1550 (89.709, 58.0271) -> (89.6742, 58.0298) projected
  line L1551 (89.6742, 58.0298) -> (89.6394, 58.0332) projected
  line L1552 (89.6394, 58.0332) -> (89.6047, 58.0371) projected
  line L1553 (89.6047, 58.0371) -> (89.5701, 58.0417) projected
  line L1554 (89.5701, 58.0417) -> (89.5356, 58.0468) projected
  line L1555 (89.5356, 58.0468) -> (89.5012, 58.0526) projected
  line L1556 (89.5012, 58.0526) -> (89.4669, 58.059) projected
  line L1557 (89.4669, 58.059) -> (89.4327, 58.0659) projected
  line L1558 (89.4327, 58.0659) -> (89.3986, 58.0735) projected
  line L1559 (89.3986, 58.0735) -> (89.3646, 58.0816) projected
  line L1560 (89.3646, 58.0816) -> (89.3308, 58.0904) projected
  line L1561 (89.3308, 58.0904) -> (89.2972, 58.0997) projected
  line L1562 (89.2972, 58.0997) -> (89.2637, 58.1096) projected
  line L1563 (89.2637, 58.1096) -> (89.2305, 58.1201) projected
  line L1564 (89.2305, 58.1201) -> (89.1973, 58.1312) projected
  line L1565 (89.1973, 58.1312) -> (89.1644, 58.1428) projected
  line L1566 (89.1644, 58.1428) -> (89.1317, 58.155) projected
  line L1567 (89.1317, 58.155) -> (89.0993, 58.1678) projected
  line L1568 (89.0993, 58.1678) -> (89.067, 58.1812) projected
  line L1569 (89.067, 58.1812) -> (89.035, 58.1951) projected
  line L1570 (89.035, 58.1951) -> (89.0032, 58.2096) projected
  line L1571 (89.0032, 58.2096) -> (88.9717, 58.2246) projected
  line L1572 (88.9717, 58.2246) -> (88.9405, 58.2402) projected
  line L1573 (88.9405, 58.2402) -> (88.9095, 58.2563) projected
  line L1574 (88.9095, 58.2563) -> (88.8789, 58.273) projected
  line L1575 (88.8789, 58.273) -> (88.8485, 58.2902) projected
  line L1576 (88.8485, 58.2902) -> (88.8184, 58.3079) projected
  line L1577 (88.8184, 58.3079) -> (88.7886, 58.3261) projected
  line L1578 (88.7886, 58.3261) -> (88.7592, 58.3449) projected
  line L1579 (88.7592, 58.3449) -> (88.7301, 58.3641) projected
  line L1580 (88.7301, 58.3641) -> (88.7013, 58.3839) projected
  line L1581 (88.7013, 58.3839) -> (88.6729, 58.4042) projected
  line L1582 (88.6729, 58.4042) -> (88.6449, 58.4249) projected
  line L1583 (88.6449, 58.4249) -> (88.6172, 58.4462) projected
  line L1584 (88.6172, 58.4462) -> (88.5898, 58.4679) projected
  line L1585 (88.5898, 58.4679) -> (88.5629, 58.4901) projected
  line L1586 (88.5629, 58.4901) -> (88.5364, 58.5128) projected
  line L1587 (88.5364, 58.5128) -> (88.5102, 58.5359) projected
  line L1588 (88.5102, 58.5359) -> (88.4845, 58.5595) projected
  line L1589 (88.4845, 58.5595) -> (88.4592, 58.5835) projected
  line L1590 (88.4592, 58.5835) -> (88.4343, 58.608) projected
  line L1591 (88.4343, 58.608) -> (88.4098, 58.6329) projected
  line L1592 (88.4098, 58.6329) -> (88.3858, 58.6582) projected
  line L1593 (88.3858, 58.6582) -> (88.3622, 58.6839) projected
  line L1594 (88.3622, 58.6839) -> (88.3391, 58.7101) projected
  line L1595 (88.3391, 58.7101) -> (88.3164, 58.7366) projected
  line L1596 (88.3164, 58.7366) -> (88.2942, 58.7636) projected
  line L1597 (88.2942, 58.7636) -> (88.2725, 58.7909) projected
  line L1598 (88.2725, 58.7909) -> (88.2512, 58.8186) projected
  line L1599 (88.2512, 58.8186) -> (88.2305, 58.8466) projected
  line L1600 (88.2305, 58.8466) -> (88.2102, 58.8751) projected
  line L1601 (88.2102, 58.8751) -> (88.1904, 58.9038) projected
  line L1602 (88.1904, 58.9038) -> (88.1711, 58.9329) projected
  line L1603 (88.1711, 58.9329) -> (88.1524, 58.9624) projected
  line L1604 (88.1524, 58.9624) -> (88.1342, 58.9921) projected
  line L1605 (88.1342, 58.9921) -> (88.1164, 59.0222) projected
  line L1606 (88.1164, 59.0222) -> (88.0992, 59.0526) projected
  line L1607 (88.0992, 59.0526) -> (88.0826, 59.0833) projected
  line L1608 (88.0826, 59.0833) -> (88.0665, 59.1142) projected
  line L1609 (88.0665, 59.1142) -> (88.0509, 59.1455) projected
  line L1610 (88.0509, 59.1455) -> (88.0359, 59.177) projected
  line L1611 (88.0359, 59.177) -> (88.0214, 59.2087) projected
  line L1612 (88.0214, 59.2087) -> (88.0075, 59.2407) projected
  line L1613 (88.0075, 59.2407) -> (87.9941, 59.273) projected
  line L1614 (87.9941, 59.273) -> (87.9813, 59.3055) projected
  line L1615 (87.9813, 59.3055) -> (87.9691, 59.3382) projected
  line L1616 (87.9691, 59.3382) -> (87.9575, 59.3711) projected
  line L1617 (87.9575, 59.3711) -> (87.9464, 59.4042) projected
  line L1618 (87.9464, 59.4042) -> (87.9359, 59.4375) projected
  line L1619 (87.9359, 59.4375) -> (87.926, 59.4709) projected
  line L1620 (87.926, 59.4709) -> (87.9166, 59.5046) projected
  line L1621 (87.9166, 59.5046) -> (87.9079, 59.5384) projected
  line L1622 (87.9079, 59.5384) -> (87.8997, 59.5723) projected
  line L1623 (87.8997, 59.5723) -> (87.8922, 59.6064) projected
  line L1624 (87.8922, 59.6064) -> (87.8852, 59.6406) projected
  line L1625 (87.8852, 59.6406) -> (87.8789, 59.6749) projected
  line L1626 (87.8789, 59.6749) -> (87.8731, 59.7093) projected
  line L1627 (87.8731, 59.7093) -> (87.868, 59.7439) projected
  line L1628 (87.868, 59.7439) -> (87.8634, 59.7785) projected
  line L1629 (87.8634, 59.7785) -> (87.8594, 59.8131) projected
  line L1630 (87.8594, 59.8131) -> (87.8561, 59.8479) projected
  line L1631 (87.8561, 59.8479) -> (87.8534, 59.8827) projected
  line L1632 (87.8534, 59.8827) -> (87.8512, 59.9175) projected
  line L1633 (87.8512, 59.9175) -> (87.8497, 59.9524) projected
  line L1634 (87.8497, 59.9524) -> (87.8488, 59.9873) projected
  line L1635 (87.8488, 59.9873) -> (87.8485, 60.0222) projected
  line L1636 (87.8485, 60.0222) -> (87.8488, 60.0571) projected
  line L1637 (87.8488, 60.0571) -> (87.8497, 60.092) projected
  line L1638 (87.8497, 60.092) -> (87.8512, 60.1269) projected
  line L1639 (87.8512, 60.1269) -> (87.8534, 60.1617) projected
  line L1640 (87.8534, 60.1617) -> (87.8561, 60.1965) projected
  line L1641 (87.8561, 60.1965) -> (87.8594, 60.2313) projected
  line L1642 (87.8594, 60.2313) -> (87.8634, 60.2659) projected
  line L1643 (87.8634, 60.2659) -> (87.868, 60.3005) projected
  line L1644 (87.868, 60.3005) -> (87.8731, 60.3351) projected
  line L1645 (87.8731, 60.3351) -> (87.8789, 60.3695) projected
  line L1646 (87.8789, 60.3695) -> (87.8852, 60.4038) projected
  line L1647 (87.8852, 60.4038) -> (87.8922, 60.438) projected
  line L1648 (87.8922, 60.438) -> (87.8997, 60.4721) projected
  line L1649 (87.8997, 60.4721) -> (87.9079, 60.506) projected
  line L1650 (87.9079, 60.506) -> (87.9166, 60.5398) projected
  line L1651 (87.9166, 60.5398) -> (87.926, 60.5735) projected
  line L1652 (87.926, 60.5735) -> (87.9359, 60.6069) projected
  line L1653 (87.9359, 60.6069) -> (87.9464, 60.6402) projected
  line L1654 (87.9464, 60.6402) -> (87.9575, 60.6733) projected
  line L1655 (87.9575, 60.6733) -> (87.9691, 60.7062) projected
  line L1656 (87.9691, 60.7062) -> (87.9813, 60.7389) projected
  line L1657 (87.9813, 60.7389) -> (87.9941, 60.7714) projected
  line L1658 (87.9941, 60.7714) -> (88.0075, 60.8037) projected
  line L1659 (88.0075, 60.8037) -> (88.0214, 60.8357) projected
  line L1660 (88.0214, 60.8357) -> (88.0359, 60.8674) projected
  line L1661 (88.0359, 60.8674) -> (88.0509, 60.8989) projected
  line L1662 (88.0509, 60.8989) -> (88.0665, 60.9302) projected
  line L1663 (88.0665, 60.9302) -> (88.0826, 60.9611) projected
  line L1664 (88.0826, 60.9611) -> (88.0992, 60.9918) projected
  line L1665 (88.0992, 60.9918) -> (88.1164, 61.0222) projected
  line L1666 (88.1164, 61.0222) -> (88.1342, 61.0523) projected
  line L1667 (88.1342, 61.0523) -> (88.1524, 61.082) projected
  line L1668 (88.1524, 61.082) -> (88.1711, 61.1115) projected
  line L1669 (88.1711, 61.1115) -> (88.1904, 61.1406) projected
  line L1670 (88.1904, 61.1406) -> (88.2102, 61.1694) projected
  line L1671 (88.2102, 61.1694) -> (88.2305, 61.1978) projected
  line L1672 (88.2305, 61.1978) -> (88.2512, 61.2258) projected
  line L1673 (88.2512, 61.2258) -> (88.2725, 61.2535) projected
  line L1674 (88.2725, 61.2535) -> (88.2942, 61.2808) projected
  line L1675 (88.2942, 61.2808) -> (88.3164, 61.3078) projected
  line L1676 (88.3164, 61.3078) -> (88.3391, 61.3343) projected
  line L1677 (88.3391, 61.3343) -> (88.3622, 61.3605) projected
  line L1678 (88.3622, 61.3605) -> (88.3858, 61.3862) projected
  line L1679 (88.3858, 61.3862) -> (88.4098, 61.4115) projected
  line L1680 (88.4098, 61.4115) -> (88.4343, 61.4364) projected
  line L1681 (88.4343, 61.4364) -> (88.4592, 61.4609) projected
  line L1682 (88.4592, 61.4609) -> (88.4845, 61.4849) projected
  line L1683 (88.4845, 61.4849) -> (88.5102, 61.5085) projected
  line L1684 (88.5102, 61.5085) -> (88.5364, 61.5316) projected
  line L1685 (88.5364, 61.5316) -> (88.5629, 61.5543) projected
  line L1686 (88.5629, 61.5543) -> (88.5898, 61.5765) projected
  line L1687 (88.5898, 61.5765) -> (88.6172, 61.5982) projected
  line L1688 (88.6172, 61.5982) -> (88.6449, 61.6195) projected
  line L1689 (88.6449, 61.6195) -> (88.6729, 61.6402) projected
  line L1690 (88.6729, 61.6402) -> (88.7013, 61.6605) projected
  line L1691 (88.7013, 61.6605) -> (88.7301, 61.6803) projected
  line L1692 (88.7301, 61.6803) -> (88.7592, 61.6995) projected
  line L1693 (88.7592, 61.6995) -> (88.7886, 61.7183) projected
  line L1694 (88.7886, 61.7183) -> (88.8184, 61.7365) projected
  line L1695 (88.8184, 61.7365) -> (88.8485, 61.7543) projected
  line L1696 (88.8485, 61.7543) -> (88.8789, 61.7714) projected
  line L1697 (88.8789, 61.7714) -> (88.9095, 61.7881) projected
  line L1698 (88.9095, 61.7881) -> (88.9405, 61.8042) projected
  line L1699 (88.9405, 61.8042) -> (88.9717, 61.8198) projected
  line L1700 (88.9717, 61.8198) -> (89.0032, 61.8348) projected
  line L1701 (89.0032, 61.8348) -> (89.035, 61.8493) projected
  line L1702 (89.035, 61.8493) -> (89.067, 61.8632) projected
  line L1703 (89.067, 61.8632) -> (89.0993, 61.8766) projected
  line L1704 (89.0993, 61.8766) -> (89.1317, 61.8894) projected
  line L1705 (89.1317, 61.8894) -> (89.1644, 61.9016) projected
  line L1706 (89.1644, 61.9016) -> (89.1973, 61.9132) projected
  line L1707 (89.1973, 61.9132) -> (89.2305, 61.9243) projected
  line L1708 (89.2305, 61.9243) -> (89.2637, 61.9348) projected
  line L1709 (89.2637, 61.9348) -> (89.2972, 61.9447) projected
  line L1710 (89.2972, 61.9447) -> (89.3308, 61.9541) projected
  line L1711 (89.3308, 61.9541) -> (89.3646, 61.9628) projected
  line L1712 (89.3646, 61.9628) -> (89.3986, 61.9709) projected
  line L1713 (89.3986, 61.9709) -> (89.4327, 61.9785) projected
  line L1714 (89.4327, 61.9785) -> (89.4669, 61.9855) projected
  line L1715 (89.4669, 61.9855) -> (89.5012, 61.9918) projected
  line L1716 (89.5012, 61.9918) -> (89.5356, 61.9976) projected
  line L1717 (89.5356, 61.9976) -> (89.5701, 62.0027) projected
  line L1718 (89.5701, 62.0027) -> (89.6047, 62.0073) projected
  line L1719 (89.6047, 62.0073) -> (89.6394, 62.0112) projected
  line L1720 (89.6394, 62.0112) -> (89.6742, 62.0146) projected
  line L1721 (89.6742, 62.0146) -> (89.709, 62.0173) projected
  line L1722 (89.709, 62.0173) -> (89.7438, 62.0195) projected
  line L1723 (89.7438, 62.0195) -> (89.7787, 62.021) projected
  line L1724 (89.7787, 62.021) -> (89.8136, 62.0219) projected
  line L1725 (89.8136, 62.0219) -> (89.8485, 62.0222) projected
  line L1726 (89.8485, 62.0222) -> (89.8834, 62.0219) projected
  line L1727 (89.8834, 62.0219) -> (89.9183, 62.021) projected
  line L1728 (89.9183, 62.021) -> (89.9532, 62.0195) projected
  line L1729 (89.9532, 62.0195) -> (89.988, 62.0173) projected
  line L1730 (89.988, 62.0173) -> (90.0228, 62.0146) projected
  line L1731 (90.0228, 62.0146) -> (90.0575, 62.0112) projected
  line L1732 (90.0575, 62.0112) -> (90.0922, 62.0073) projected
  line L1733 (90.0922, 62.0073) -> (90.1268, 62.0027) projected
  line L1734 (90.1268, 62.0027) -> (90.1614, 61.9976) projected
  line L1735 (90.1614, 61.9976) -> (90.1958, 61.9918) projected
  line L1736 (90.1958, 61.9918) -> (90.2301, 61.9855) projected
  line L1737 (90.2301, 61.9855) -> (90.2643, 61.9785) projected
  line L1738 (90.2643, 61.9785) -> (90.2984, 61.9709) projected
  line L1739 (90.2984, 61.9709) -> (90.3323, 61.9628) projected
  line L1740 (90.3323, 61.9628) -> (90.3661, 61.9541) projected
  line L1741 (90.3661, 61.9541) -> (90.3998, 61.9447) projected
  line L1742 (90.3998, 61.9447) -> (90.4332, 61.9348) projected
  line L1743 (90.4332, 61.9348) -> (90.4665, 61.9243) projected
  line L1744 (90.4665, 61.9243) -> (90.4996, 61.9132) projected
  line L1745 (90.4996, 61.9132) -> (90.5325, 61.9016) projected
  line L1746 (90.5325, 61.9016) -> (90.5652, 61.8894) projected
  line L1747 (90.5652, 61.8894) -> (90.5977, 61.8766) projected
  line L1748 (90.5977, 61.8766) -> (90.6299, 61.8632) projected
  line L1749 (90.6299, 61.8632) -> (90.662, 61.8493) projected
  line L1750 (90.662, 61.8493) -> (90.6937, 61.8348) projected
  line L1751 (90.6937, 61.8348) -> (90.7252, 61.8198) projected
  line L1752 (90.7252, 61.8198) -> (90.7565, 61.8042) projected
  line L1753 (90.7565, 61.8042) -> (90.7874, 61.7881) projected
  line L1754 (90.7874, 61.7881) -> (90.8181, 61.7714) projected
  line L1755 (90.8181, 61.7714) -> (90.8485, 61.7543) projected
  line L1756 (90.8485, 61.7543) -> (90.8786, 61.7365) projected
  line L1757 (90.8786, 61.7365) -> (90.9083, 61.7183) projected
  line L1758 (90.9083, 61.7183) -> (90.9378, 61.6995) projected
  line L1759 (90.9378, 61.6995) -> (90.9669, 61.6803) projected
  line L1760 (90.9669, 61.6803) -> (90.9956, 61.6605) projected
  line L1761 (90.9956, 61.6605) -> (91.0241, 61.6402) projected
  line L1762 (91.0241, 61.6402) -> (91.0521, 61.6195) projected
  line L1763 (91.0521, 61.6195) -> (91.0798, 61.5982) projected
  line L1764 (91.0798, 61.5982) -> (91.1071, 61.5765) projected
  line L1765 (91.1071, 61.5765) -> (91.1341, 61.5543) projected
  line L1766 (91.1341, 61.5543) -> (91.1606, 61.5316) projected
  line L1767 (91.1606, 61.5316) -> (91.1867, 61.5085) projected
  line L1768 (91.1867, 61.5085) -> (91.2125, 61.4849) projected
  line L1769 (91.2125, 61.4849) -> (91.2378, 61.4609) projected
  line L1770 (91.2378, 61.4609) -> (91.2627, 61.4364) projected
  line L1771 (91.2627, 61.4364) -> (91.2872, 61.4115) projected
  line L1772 (91.2872, 61.4115) -> (91.3112, 61.3862) projected
  line L1773 (91.3112, 61.3862) -> (91.3348, 61.3605) projected
  line L1774 (91.3348, 61.3605) -> (91.3579, 61.3343) projected
  line L1775 (91.3579, 61.3343) -> (91.3806, 61.3078) projected
  line L1776 (91.3806, 61.3078) -> (91.4028, 61.2808) projected
  line L1777 (91.4028, 61.2808) -> (91.4245, 61.2535) projected
  line L1778 (91.4245, 61.2535) -> (91.4458, 61.2258) projected
  line L1779 (91.4458, 61.2258) -> (91.4665, 61.1978) projected
  line L1780 (91.4665, 61.1978) -> (91.4868, 61.1694) projected
  line L1781 (91.4868, 61.1694) -> (91.5066, 61.1406) projected
  line L1782 (91.5066, 61.1406) -> (91.5258, 61.1115) projected
  line L1783 (91.5258, 61.1115) -> (91.5446, 61.082) projected
  line L1784 (91.5446, 61.082) -> (91.5628, 61.0523) projected
  line L1785 (91.5628, 61.0523) -> (91.5805, 61.0222) projected
  line L1786 (91.5805, 61.0222) -> (91.5977, 60.9918) projected
  line L1787 (91.5977, 60.9918) -> (91.6144, 60.9611) projected
  line L1788 (91.6144, 60.9611) -> (91.6305, 60.9302) projected
  line L1789 (91.6305, 60.9302) -> (91.6461, 60.8989) projected
  line L1790 (91.6461, 60.8989) -> (91.6611, 60.8674) projected
  line L1791 (91.6611, 60.8674) -> (91.6756, 60.8357) projected
  line L1792 (91.6756, 60.8357) -> (91.6895, 60.8037) projected
  line L1793 (91.6895, 60.8037) -> (91.7028, 60.7714) projected
  line L1794 (91.7028, 60.7714) -> (91.7156, 60.7389) projected
  line L1795 (91.7156, 60.7389) -> (91.7279, 60.7062) projected
  line L1796 (91.7279, 60.7062) -> (91.7395, 60.6733) projected
  line L1797 (91.7395, 60.6733) -> (91.7506, 60.6402) projected
  line L1798 (91.7506, 60.6402) -> (91.7611, 60.6069) projected
  line L1799 (91.7611, 60.6069) -> (91.771, 60.5735) projected
  line L1800 (91.771, 60.5735) -> (91.7803, 60.5398) projected
  line L1801 (91.7803, 60.5398) -> (91.7891, 60.506) projected
  line L1802 (91.7891, 60.506) -> (91.7972, 60.4721) projected
  line L1803 (91.7972, 60.4721) -> (91.8048, 60.438) projected
  line L1804 (91.8048, 60.438) -> (91.8117, 60.4038) projected
  line L1805 (91.8117, 60.4038) -> (91.8181, 60.3695) projected
  line L1806 (91.8181, 60.3695) -> (91.8239, 60.3351) projected
  line L1807 (91.8239, 60.3351) -> (91.829, 60.3005) projected
  line L1808 (91.829, 60.3005) -> (91.8336, 60.2659) projected
  line L1809 (91.8336, 60.2659) -> (91.8375, 60.2313) projected
  line L1810 (91.8375, 60.2313) -> (91.8409, 60.1965) projected
  line L1811 (91.8409, 60.1965) -> (91.8436, 60.1617) projected
  line L1812 (91.8436, 60.1617) -> (91.8457, 60.1269) projected
  line L1813 (91.8457, 60.1269) -> (91.8473, 60.092) projected
  line L1814 (91.8473, 60.092) -> (91.8482, 60.0571) projected
  line L1815 (91.8482, 60.0571) -> (91.8485, 60.0222) projected
  line L1816 (91.8485, -59.9778) -> (91.8482, -60.0127) projected
  line L1817 (91.8482, -60.0127) -> (91.8473, -60.0476) projected
  line L1818 (91.8473, -60.0476) -> (91.8457, -60.0825) projected
  line L1819 (91.8457, -60.0825) -> (91.8436, -60.1173) projected
  line L1820 (91.8436, -60.1173) -> (91.8409, -60.1521) projected
  line L1821 (91.8409, -60.1521) -> (91.8375, -60.1869) projected